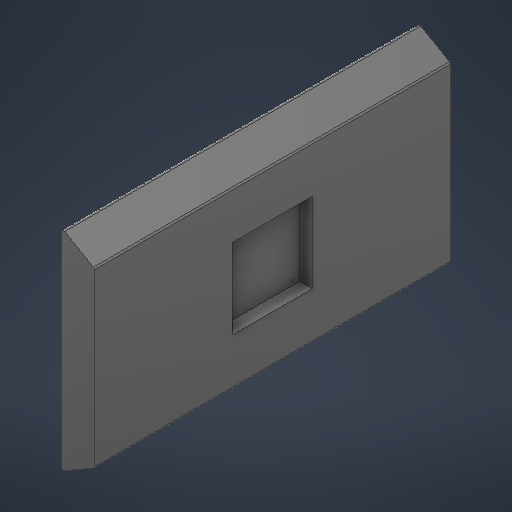
# Autodesk Inventor part: Monitor v1.0
Saved by Autodesk Inventor 2027 (Build 310192060, 192F)
## iProperties
Created: 2026-05-21
Part Number: Monitor v1.0
Material: Generic
Document SubType Name: Modeling
Designer: cheap
Density: 1 g/cm^3
Appearance: Default
Author: cheap
Autodesk Inventor part; units mm, degrees
ref_plane "YZ Plane" through (0, 0, 0) normal (1, 0, 0) x (0, 1, 0)
ref_plane "XZ Plane" through (0, 0, 0) normal (0, 1, 0) x (-1, 0, 0)
ref_plane "XY Plane" through (0, 0, 0) normal (0, 0, 1) x (1, 0, 0)
sketch "Sketch1" plane through (0, 0, 0) normal (0, 0, 1) x (1, 0, 0)
  line L0 (0, 5.4993) -> (0, 312.0007)
  line L1 (4.7625, 314.7504) -> (47.9059, 289.8415)
  line L2 (0, 158.75) -> (212.725, 158.75) construction
  line L3 (4.7625, 2.7496) -> (47.9059, 27.6585)
  line L4 (49.4934, 287.0919) -> (49.4934, 30.4081)
  arc A0 (49.4934, 287.0919) -> (47.9059, 289.8415) centre (46.3184, 287.0919) ccw
  arc A1 (47.9059, 27.6585) -> (49.4934, 30.4081) centre (46.3184, 30.4081) ccw
  arc A2 (0, 5.4993) -> (4.7625, 2.7496) centre (3.175, 5.4993) ccw
  arc A3 (4.7625, 314.7504) -> (0, 312.0007) centre (3.175, 312.0007) ccw
  point P0 (0, 0)
  point P1 (0, 317.5)
  point P2 (49.4934, 288.925)
  point P3 (49.4934, 28.575)
  dimension "d0" = 317.5
  dimension "d1" = 57.15
  dimension "d2" = 60
  dimension "d3" = 3.175
  dimension "d4" = 3.175
  constraints: 10 end point, 8 point on circle, 8 point on line, 8 tangent, 4 centre point, 2 equal radius, 2 vertical, 1 horizontal, 1 midpoint, 1 symmetric about line
  measures "d0" distance of point (0, 0) point (0, 317.5)
  measures "d1" distance of point (0, 317.5) point (49.493, 288.925)
  measures "d2" angle of L0 L1
  measures "d3" radius of A0
  measures "d4" radius of A2
extrude "Extrusion1" add sketch "Sketch1" along normal blind 536.575
sketch "Sketch4" plane through (49.4934, 30.4081, 0) normal (1, 0, 0) x (0, 0, -1)
  line L0 (-536.575, 0) -> (-536.575, 256.6838) construction
  line L1 (-536.575, 128.3419) -> (0, 128.3419) construction
  line L2 (0, 0) -> (0, 256.6838) construction
  line L3 (0, 256.6838) -> (-536.575, 256.6838) construction
  line L4 (-268.2875, 256.6838) -> (-268.2875, 0) construction
  line L5 (0, 0) -> (-536.575, 0) construction
  line L6 (-328.6125, 188.6669) -> (-207.9625, 188.6669)
  line L7 (-207.9625, 188.6669) -> (-207.9625, 68.0169)
  line L8 (-207.9625, 68.0169) -> (-328.6125, 68.0169)
  line L9 (-328.6125, 68.0169) -> (-328.6125, 188.6669)
  line L10 (-328.6125, 188.6669) -> (-207.9625, 68.0169) construction
  line L11 (-207.9625, 188.6669) -> (-328.6125, 68.0169) construction
  point P0 (0, -30.4081)
  point P1 (-268.2875, 128.3419)
  dimension "d9" = 120.65
  dimension "d10" = 120.65
  constraints: 16 end point, 7 midpoint, 2 parallel, 1 horizontal, 1 perpendicular
  measures "d9" distance of L7.end L8.end
  measures "d10" distance of L6.end L7.end
extrude "Extrusion2" cut sketch "Sketch4" against normal blind 19.05
sketch "Sketch5" plane through (30.4434, 30.4081, 0) normal (1, 0, 0) x (0, 0, -1)
  circle A0 centre (-218.6305, 175.9669) radius 1.5875
  circle A1 centre (-320.2305, 175.9669) radius 1.5875
  circle A2 centre (-218.6305, 74.3669) radius 1.5875
  circle A3 centre (-320.2305, 74.3669) radius 1.5875
  line L0 (-328.6125, 68.0169) -> (-328.6125, 188.6669) projected
  line L1 (-207.9625, 68.0169) -> (-328.6125, 68.0169) projected
  line L2 (-320.2305, 175.9669) -> (-218.6305, 175.9669) construction
  line L3 (-218.6305, 175.9669) -> (-218.6305, 74.3669) construction
  line L4 (-218.6305, 74.3669) -> (-320.2305, 74.3669) construction
  line L5 (-320.2305, 74.3669) -> (-320.2305, 175.9669) construction
  point P0 (0, -30.4081)
  dimension "d13" = 3.175
  dimension "d14" = 3.175
  dimension "d15" = 3.175
  dimension "d16" = 101.6
  dimension "d17" = 101.6
  dimension "d18" = 101.6
  dimension "d19" = 8.382
  dimension "d20" = 8.382
  dimension "d21" = 107.95
  constraints: 8 end point, 4 centre point, 2 perpendicular
  measures "d13" diameter of A0
  measures "d14" diameter of A1
  measures "d15" diameter of A2
  measures "d16" distance of L2.end L2.start
  measures "d17" distance of L3.end L4.end
  measures "d18" distance of L4.end L2.start
  measures "d19" distance from line of L2.start L0
  measures "d20" distance from line of L0 L4.end
  measures "d21" distance from line of L1 L2.start
extrude "Extrusion3" cut sketch "Sketch5" against normal blind 12.7
sketch "Sketch6" plane through (0, 5.4993, 0) normal (-1, 0, 0) x (0, 0, 1)
  line L0 (0, 306.5015) -> (0, 0) construction
  line L1 (0, 153.2507) -> (536.575, 153.2507) construction
  line L2 (536.575, 24.9088) -> (536.575, 281.5927) construction
  line L3 (0, 309.6765) -> (536.575, 309.6765) construction
  line L4 (0, 0) -> (536.575, 0) construction
  line L5 (0, -3.175) -> (536.575, -3.175) construction
  line L6 (268.2875, -3.175) -> (268.2875, 309.6765) construction
  line L7 (11.1125, 296.1257) -> (525.4625, 296.1257)
  line L8 (525.4625, 296.1257) -> (525.4625, 10.3757)
  line L9 (525.4625, 10.3757) -> (11.1125, 10.3757)
  line L10 (11.1125, 10.3757) -> (11.1125, 296.1257)
  line L11 (11.1125, 296.1257) -> (525.4625, 10.3757) construction
  line L12 (525.4625, 296.1257) -> (11.1125, 10.3757) construction
  point P0 (0, -5.4993)
  point P1 (268.2875, 153.2507)
  dimension "d24" = 285.75
  constraints: 16 end point, 7 midpoint, 2 parallel, 1 horizontal, 1 perpendicular
  measures "d24" distance of L7.end L8.end
extrude "Extrusion4" cut sketch "Sketch6" against normal blind 3.175
body "Solid1"
